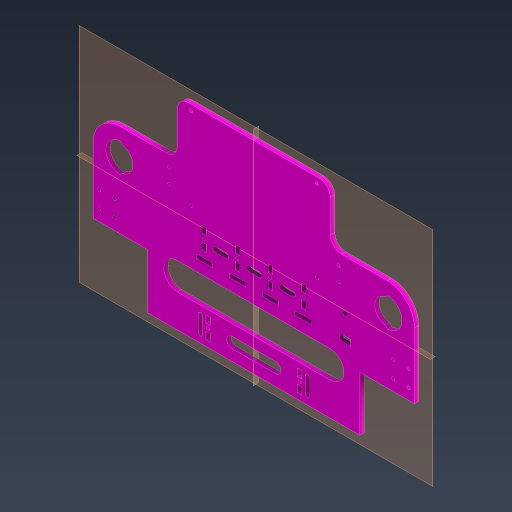
# Autodesk Inventor part: Передняя_крышка
Saved by Autodesk Inventor 2023.2 (Build 272271030, 271C)
## iProperties
Created: 2025-12-12
Part Number: Передняя_крышка
Material: Типовые
Document SubType Name: Modeling
Designer: Олег Коноваленко
Density: 1 g/cm^3
Appearance: Пурпурный
Author: Олег Коноваленко
Autodesk Inventor part; units mm, degrees
sketch "Эскиз1" plane through (0, 0, 0) normal (0, 0, 1) x (1, 0, 0)
  line L0 (-147, -42.5) -> (147, -42.5)
  line L1 (147, -42.5) -> (147, 42.5)
  line L2 (147, 42.5) -> (-147, 42.5)
  line L3 (-147, 42.5) -> (-147, -42.5)
  line L4 (-147, -42.5) -> (147, 42.5) construction
  line L5 (147, -42.5) -> (-147, 42.5) construction
  point P0 (0, 0)
  dimension "d0" = 294
  dimension "d1" = 85
  constraints: 12 end point, 2 midpoint, 2 parallel, 1 horizontal, 1 perpendicular
  measures "d0" distance of L1.end L2.end
  measures "d1" distance of L2.end L0.start
extrude "Выдавливание1" add sketch "Эскиз1" along normal mid plane 4
sketch "Эскиз5" plane through (0, 0, 2) normal (0, 0, 1) x (1, 0, 0)
  arc A0 (147, 17.5) -> (122, 42.5) centre (122, 17.5) ccw projected
  line L0 (147, -42.5) -> (147, 42.5) projected
  line L1 (147, 42.5) -> (-147, 42.5) projected
  point P0 (0, 0)
  point P1 (147, 17.5)
extrude "Выдавливание4" cut sketch "Эскиз5" against normal up to next
sketch "Эскиз6" plane through (0, 0, -2) normal (0, 0, -1) x (-1, 0, 0)
  line L0 (147, -42.5) -> (-147, -42.5) projected
  line L1 (-97, -42.5) -> (97, -42.5)
  line L2 (97, -42.5) -> (97, -92.5)
  line L3 (97, -92.5) -> (-97, -92.5)
  line L4 (-97, -92.5) -> (-97, -42.5)
  line L5 (-97, -92.5) -> (-97, -42.5) projected
  line L6 (147, -42.5) -> (147, 42.5) projected
  point P0 (0, 0)
  dimension "d18" = 50
  constraints: 8 end point, 2 parallel, 1 horizontal, 1 perpendicular, 1 point on line
  measures "d18" distance between parallel lines of L6 L2
extrude "Выдавливание5" add sketch "Эскиз6" against normal blind 4
sketch "Эскиз7" plane through (0, 0, -2) normal (0, 0, -1) x (-1, 0, 0)
  circle A0 centre (-127.5, -32.5) radius 1.6 projected
  circle A1 centre (-127.5, -17.5) radius 1.6 projected
  circle A2 centre (-141.5, -17.5) radius 1.6 projected
  circle A3 centre (-141.5, -32.5) radius 1.6 projected
  point P0 (0, 0)
extrude "Выдавливание6" cut sketch "Эскиз7" against normal up to next
sketch "Эскиз8" plane through (0, 0, -2) normal (0, 0, -1) x (-1, 0, 0)
  circle A0 centre (-122, 17.5) radius 6 projected
  circle A1 centre (-122, 17.5) radius 13.5
  point P0 (0, 0)
  dimension "d23" = 7.5
  constraints: 1 centre point
  measures "d23" radial gap between concentric circles of A1 A0
extrude "Выдавливание7" cut sketch "Эскиз8" against normal up to next contours A0 | A1
sketch "Эскиз9" plane through (0, 0, -2) normal (0, 0, -1) x (-1, 0, 0)
  circle A0 centre (-122, 17.5) radius 13.5 projected
  arc A1 (-122, 6) -> (-122, 29) centre (-122, 17.5) ccw
  line L0 (-122, 4) -> (-122, 31)
  point P0 (0, 0)
  dimension "d26" = 11.5
  constraints: 4 point on circle, 2 end point, 2 point on line, 1 centre point, 1 concentric, 1 midpoint, 1 vertical
  measures "d26" radius of A1
extrude "Выдавливание8" add sketch "Эскиз9" against normal blind 4 contours A0 L0 A1
mirror "Зеркальное отражение1" about plane through (0, 0, 0) normal (1, 0, 0) of "Выдавливание6", "Выдавливание7", "Выдавливание8", "Выдавливание4"
fillet "Сопряжение2" radius 3 4 edges at (122, 6, 0) (122, 29, 0) (-122, 29, 0) (-122, 6, 0)
sketch "Эскиз10" plane through (0, 0, -2) normal (0, 0, -1) x (-1, 0, 0)
  line L0 (70, -50) -> (-70, -50) construction
  line L1 (70, -37.5) -> (-70, -37.5)
  line L2 (-70, -62.5) -> (70, -62.5)
  arc A0 (70, -62.5) -> (70, -37.5) centre (70, -50) ccw
  arc A1 (-70, -37.5) -> (-70, -62.5) centre (-70, -50) ccw
  line L3 (0, -119.5) -> (0, 69.5) projected
  line L4 (-205.8, 0) -> (205.8, 0) projected
  point P0 (0, 0)
  point P1 (0, -50)
  dimension "d32" = 140
  dimension "d33" = 50
  dimension "d34" = 12.5
  constraints: 8 end point, 4 point on circle, 4 tangent, 2 centre point, 1 horizontal, 1 midpoint, 1 parallel, 1 point on line
  measures "d32" distance of L0.start L0.end
  measures "d33" distance between parallel lines of L4 L0
  measures "d34" distance between parallel lines of L0 L2
extrude "Выдавливание9" cut sketch "Эскиз10" against normal up to next
sketch "Эскиз11" plane through (0, 0, -2) normal (0, 0, -1) x (-1, 0, 0)
  circle A0 centre (-83.4599, -3) radius 2.5 projected
  line L0 (-78.2599, -26.63) -> (-88.6599, -26.63) projected
  line L1 (-78.2599, -20.73) -> (-78.2599, -26.63) projected
  line L2 (-88.6599, -20.73) -> (-78.2599, -20.73) projected
  line L3 (-88.6599, -20.73) -> (-88.6599, -26.63) projected
  point P0 (0, 0)
extrude "Выдавливание10" cut sketch "Эскиз11" against normal up to next
sketch "Эскиз12" plane through (0, 0, -2) normal (0, 0, -1) x (-1, 0, 0)
  line L0 (-122, 42.5) -> (122, 42.5) projected
  line L1 (70, 42.5) -> (70, 92.5)
  line L2 (70, 92.5) -> (-70, 92.5)
  line L3 (-70, 92.5) -> (-70, 42.5)
  line L4 (0, -69.5) -> (0, 119.5) construction
  point P0 (0, 0)
  point P1 (0, 92.5)
  dimension "d39" = 140
  dimension "d40" = 50
  constraints: 6 end point, 3 point on line, 2 perpendicular, 1 midpoint, 1 parallel
  measures "d39" distance of L1.end L2.end
  measures "d40" distance between parallel lines of L0 L2
extrude "Выдавливание11" add sketch "Эскиз12" against normal blind 4
sketch "Эскиз13" plane through (0, 0, 2) normal (0, 0, 1) x (1, 0, 0)
  line L0 (52.5, -23.5) -> (37.5, -23.5) projected
  line L1 (37.5, -27.5) -> (37.5, -23.5) projected
  line L2 (52.5, -27.5) -> (37.5, -27.5) projected
  line L3 (52.5, -27.5) -> (52.5, -23.5) projected
  line L4 (22.5, -23.5) -> (7.5, -23.5) projected
  line L5 (7.5, -27.5) -> (7.5, -23.5) projected
  line L6 (22.5, -27.5) -> (7.5, -27.5) projected
  line L7 (22.5, -27.5) -> (22.5, -23.5) projected
  line L8 (-7.5, -23.5) -> (-22.5, -23.5) projected
  line L9 (-22.5, -27.5) -> (-22.5, -23.5) projected
  line L10 (-7.5, -27.5) -> (-22.5, -27.5) projected
  line L11 (-7.5, -27.5) -> (-7.5, -23.5) projected
  line L12 (-37.5, -23.5) -> (-52.5, -23.5) projected
  line L13 (-52.5, -27.5) -> (-52.5, -23.5) projected
  line L14 (-37.5, -27.5) -> (-52.5, -27.5) projected
  line L15 (-37.5, -27.5) -> (-37.5, -23.5) projected
  point P0 (0, 0)
extrude "Выдавливание12" cut sketch "Эскиз13" against normal up to next
sketch "Эскиз14" plane through (0, 0, 2) normal (0, 0, 1) x (1, 0, 0)
  line L0 (47.7, -11.5) -> (47.7, -18.5) projected
  line L1 (47.7, -11.5) -> (43.7, -11.5) projected
  line L2 (43.7, -18.5) -> (43.7, -11.5) projected
  line L3 (47.7, -18.5) -> (43.7, -18.5) projected
  line L4 (47.7, -5.5) -> (43.7, -5.5) projected
  line L5 (43.7, -5.5) -> (43.7, 1.5) projected
  line L6 (47.7, 1.5) -> (47.7, -5.5) projected
  line L7 (47.7, 1.5) -> (43.7, 1.5) projected
  line L8 (17, -5.5) -> (13, -5.5) projected
  line L9 (17, 1.5) -> (17, -5.5) projected
  line L10 (17, 1.5) -> (13, 1.5) projected
  line L11 (13, -5.5) -> (13, 1.5) projected
  line L12 (17, -11.5) -> (13, -11.5) projected
  line L13 (17, -11.5) -> (17, -18.5) projected
  line L14 (13, -18.5) -> (13, -11.5) projected
  line L15 (17, -18.5) -> (13, -18.5) projected
  line L16 (-17, -5.5) -> (-17, 1.5) projected
  line L17 (-13, 1.5) -> (-13, -5.5) projected
  line L18 (-13, 1.5) -> (-17, 1.5) projected
  line L19 (-13, -5.5) -> (-17, -5.5) projected
  line L20 (-13, -11.5) -> (-17, -11.5) projected
  line L21 (-13, -11.5) -> (-13, -18.5) projected
  line L22 (-17, -18.5) -> (-17, -11.5) projected
  line L23 (-13, -18.5) -> (-17, -18.5) projected
  line L24 (-43.7, 1.5) -> (-47.7, 1.5) projected
  line L25 (-43.7, 1.5) -> (-43.7, -5.5) projected
  line L26 (-47.7, -5.5) -> (-47.7, 1.5) projected
  line L27 (-43.7, -5.5) -> (-47.7, -5.5) projected
  line L28 (-43.7, -11.5) -> (-47.7, -11.5) projected
  line L29 (-43.7, -11.5) -> (-43.7, -18.5) projected
  line L30 (-47.7, -18.5) -> (-47.7, -11.5) projected
  line L31 (-43.7, -18.5) -> (-47.7, -18.5) projected
  circle A0 centre (45.7, -8.5) radius 1.5
  circle A1 centre (15, -8.5) radius 1.5
  circle A2 centre (-15, -8.5) radius 1.5
  circle A3 centre (-45.7, -8.5) radius 1.5
  line L32 (-45.7, -10.8) -> (-45.7, 50.8) construction
  line L33 (-15, -10.8) -> (-15, 50.8) construction
  line L34 (15, -10.8) -> (15, 50.8) construction
  line L35 (45.7, -10.8) -> (45.7, 50.8) construction
  point P0 (0, 0)
  point P1 (46.5, 12)
  point P2 (-15.8, 12)
  point P3 (44.9, -11)
  point P4 (14.2, -1)
  point P5 (-15.8, -11)
  point P6 (-44.9, -11)
  point P7 (-44.9, 2)
  dimension "d47" = 3
  dimension "d48" = 3
  dimension "d49" = 3
  dimension "d50" = 3
  dimension "d51" = 3
  constraints: 8 end point, 4 centre point, 4 point on line, 4 vertical, 3 equal radius, 8 other
  measures "d47" distance from line of L4 A0.centre
  measures "d48" distance from line of L8 A1.centre
  measures "d49" distance from line of L19 A2.centre
  measures "d50" distance from line of L27 A3.centre
  measures "d51" diameter of A0
extrude "Выдавливание13" cut sketch "Эскиз14" against normal up to next
fillet "Сопряжение5" radius 10 2 edges at (-70, 92.5, 0) (70, 92.5, 0)
sketch "Эскиз15" plane through (0, 0, -2) normal (0, 0, -1) x (-1, 0, 0)
  circle A0 centre (57.5, 12.25) radius 1.5 projected
  circle A1 centre (-57.5, 12.25) radius 1.5 projected
  circle A2 centre (-57.5, 87.25) radius 1.5 projected
  circle A3 centre (57.5, 87.25) radius 1.5 projected
  point P0 (0, 0)
extrude "Выдавливание14" cut sketch "Эскиз15" against normal up to next
sketch "Эскиз16" plane through (0, 0, -2) normal (0, 0, -1) x (-1, 0, 0)
  line L0 (20, -77.5) -> (-20, -77.5) construction
  line L1 (20, -72.5) -> (-20, -72.5)
  line L2 (-20, -82.5) -> (20, -82.5)
  arc A0 (20, -82.5) -> (20, -72.5) centre (20, -77.5) ccw
  arc A1 (-20, -72.5) -> (-20, -82.5) centre (-20, -77.5) ccw
  line L3 (0, -129.5) -> (0, 129.5) projected
  line L4 (70, -62.5) -> (-70, -62.5) projected
  point P0 (0, 0)
  point P1 (0, -77.5)
  dimension "d57" = 40
  dimension "d58" = 15
  dimension "d59" = 5
  constraints: 8 end point, 4 point on circle, 4 tangent, 2 centre point, 1 horizontal, 1 midpoint, 1 parallel, 1 point on line
  measures "d57" distance of L0.start L0.end
  measures "d58" distance between parallel lines of L4 L0
  measures "d59" distance between parallel lines of L0 L2
extrude "Выдавливание15" cut sketch "Эскиз16" against normal up to next
sketch "Эскиз17" plane through (0, 0, 2) normal (0, 0, 1) x (1, 0, 0)
  line L0 (44, -80.5) -> (40, -80.5) projected
  line L1 (40, -87.5) -> (40, -80.5) projected
  line L2 (44, -87.5) -> (40, -87.5) projected
  line L3 (44, -80.5) -> (44, -87.5) projected
  line L4 (44, -67.5) -> (40, -67.5) projected
  line L5 (40, -74.5) -> (40, -67.5) projected
  line L6 (44, -74.5) -> (40, -74.5) projected
  line L7 (44, -67.5) -> (44, -74.5) projected
  line L8 (-40, -80.5) -> (-44, -80.5) projected
  line L9 (-44, -87.5) -> (-44, -80.5) projected
  line L10 (-40, -87.5) -> (-44, -87.5) projected
  line L11 (-40, -80.5) -> (-40, -87.5) projected
  line L12 (-40, -67.5) -> (-44, -67.5) projected
  line L13 (-44, -74.5) -> (-44, -67.5) projected
  line L14 (-40, -74.5) -> (-44, -74.5) projected
  line L15 (-40, -67.5) -> (-40, -74.5) projected
  line L16 (42, -103.3) -> (42, -55.7) construction
  line L17 (-42, -103.3) -> (-42, -55.7) construction
  circle A0 centre (-42, -77.5) radius 1.5
  circle A1 centre (42, -77.5) radius 1.5
  point P0 (0, 0)
  dimension "d62" = 3
  dimension "d63" = 3
  dimension "d64" = 3
  constraints: 4 end point, 2 centre point, 2 point on line, 2 vertical, 1 equal radius, 4 other
  measures "d62" diameter of A1
  measures "d63" distance from line of L0 A1.centre
  measures "d64" distance from line of L8 A0.centre
extrude "Выдавливание16" cut sketch "Эскиз17" against normal up to next
sketch "Эскиз18" plane through (0, 0, -2) normal (0, 0, -1) x (-1, 0, 0)
  line L0 (-49, -85) -> (-49, -70) construction
  line L1 (-47, -85) -> (-47, -70)
  line L2 (-51, -70) -> (-51, -85)
  arc A0 (-51, -85) -> (-47, -85) centre (-49, -85) ccw
  arc A1 (-47, -70) -> (-51, -70) centre (-49, -70) ccw
  line L3 (70, -62.5) -> (-70, -62.5) projected
  line L4 (-42, -55.7) -> (-42, -103.3)
  point P0 (0, 0)
  point P1 (-49, -77.5)
  dimension "d67" = 15
  dimension "d68" = 2
  dimension "d69" = 15
  dimension "d70" = 7
  constraints: 10 end point, 4 point on circle, 4 tangent, 2 centre point, 2 vertical, 1 midpoint, 1 parallel, 2 other
  measures "d67" distance of L0.start L0.end
  measures "d68" distance from line of L2 point (-49, -77.5)
  measures "d69" distance from line of L3 point (-49, -77.5)
  measures "d70" distance from line of point (-49, -77.5) L4
extrude "Выдавливание17" cut sketch "Эскиз18" against normal up to next
mirror "Зеркальное отражение2" about plane through (0, 0, 0) normal (1, 0, 0) of "Выдавливание17"
sketch "Эскиз19" plane through (0, 0, 2) normal (0, 0, 1) x (1, 0, 0)
  circle A0 centre (-80, 52.5) radius 10
  line L0 (-70, 82.5) -> (-70, 42.5) projected
  line L1 (-70, 42.5) -> (-122, 42.5) projected
  line L2 (70, 42.5) -> (70, 82.5) projected
  line L3 (122, 42.5) -> (70, 42.5) projected
  circle A1 centre (80, 52.5) radius 10
  point P0 (0, 0)
  point P1 (80, 42.5)
  point P2 (70, 52.5)
  point P3 (-80, 42.5)
  point P4 (-70, 52.5)
  dimension "d73" = 20
  constraints: 4 tangent, 2 centre point, 1 equal radius
  measures "d73" diameter of A0
extrude "Выдавливание18" add sketch "Эскиз19" against normal up to surface (4 mm away) contours L0 L1 A0 | L2 A1 L3
sketch "Эскиз20" plane through (0, 0, -2) normal (0, 0, -1) x (-1, 0, 0)
  circle A0 centre (77.5, 19.25) radius 1.5 projected
  circle A1 centre (77.5, 32.25) radius 1.5 projected
  circle A2 centre (-77.5, 19.25) radius 1.5 projected
  circle A3 centre (-77.5, 32.25) radius 1.5 projected
  point P0 (0, 0)
extrude "Выдавливание19" cut sketch "Эскиз20" against normal up to next
sketch "Эскиз22" plane through (0, 0, -2) normal (0, 0, -1) x (-1, 0, 0)
  line L0 (35.35, -11.5) -> (25.35, -11.5) construction
  line L1 (35.35, -9) -> (25.35, -9)
  line L2 (25.35, -14) -> (35.35, -14)
  arc A0 (35.35, -14) -> (35.35, -9) centre (35.35, -11.5) ccw
  arc A1 (25.35, -9) -> (25.35, -14) centre (25.35, -11.5) ccw
  line L3 (43.7, -18.5) -> (43.7, -11.5) projected
  line L4 (52.5, -27.5) -> (37.5, -27.5) projected
  line L5 (5, -11.5) -> (-5, -11.5) construction
  line L6 (5, -9) -> (-5, -9)
  line L7 (-5, -14) -> (5, -14)
  arc A2 (5, -14) -> (5, -9) centre (5, -11.5) ccw
  arc A3 (-5, -9) -> (-5, -14) centre (-5, -11.5) ccw
  line L8 (-25.35, -11.5) -> (-35.35, -11.5) construction
  line L9 (-25.35, -9) -> (-35.35, -9)
  line L10 (-35.35, -14) -> (-25.35, -14)
  arc A4 (-25.35, -14) -> (-25.35, -9) centre (-25.35, -11.5) ccw
  arc A5 (-35.35, -9) -> (-35.35, -14) centre (-35.35, -11.5) ccw
  line L11 (0, -129.5) -> (0, 129.5) projected
  point P0 (0, 0)
  point P1 (30.35, -11.5)
  point P2 (0, -11.5)
  point P3 (-30.35, -11.5)
  point P4 (0, -11.5)
  dimension "d84" = 2.5
  dimension "d85" = 10
  dimension "d86" = 13.35
  dimension "d87" = 16
  dimension "d90" = 30.35
  constraints: 24 end point, 12 point on circle, 6 centre point, 4 tangent, 2 horizontal, 2 midpoint, 1 collinear, 1 parallel, 23 other
  measures "d84" distance between parallel lines of L0 L2
  measures "d85" distance of L0.start L0.end
  measures "d86" distance from line of L3 point (30.35, -11.5)
  measures "d87" distance from line of L4 point (30.35, -11.5)
  measures "d90" distance of L1.start L6.start
extrude "Выдавливание21" cut sketch "Эскиз22" against normal up to next
